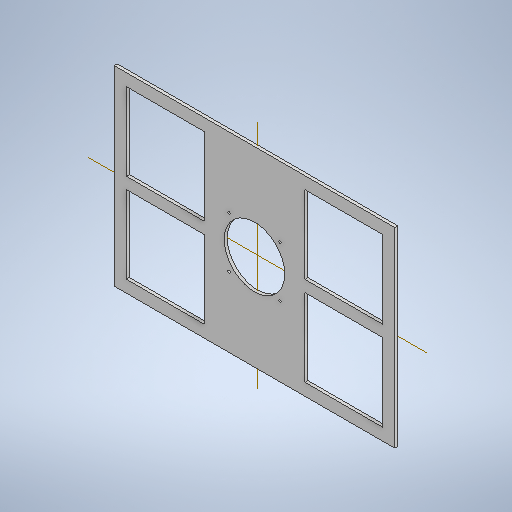
# Autodesk Inventor part: 가로세로
Saved by Autodesk Inventor 2025.1 (Build 291241000, 241)
## iProperties
Created: 2024-10-28
Part Number: 가로세로
Material: 일반
Document SubType Name: Modeling
Designer: gmsee
Density: 1 g/cm^3
Appearance: 기본값
Author: gmsee
Autodesk Inventor part; units mm, degrees
ref_plane "YZ Plane" through (0, 0, 0) normal (1, 0, 0) x (0, 1, 0)
ref_plane "XZ Plane" through (0, 0, 0) normal (0, 1, 0) x (-1, 0, 0)
ref_plane "XY Plane" through (0, 0, 0) normal (0, 0, 1) x (1, 0, 0)
sketch "스케치3" plane through (0, 0, 0) normal (0, 0, 1) x (1, 0, 0)
  line L0 (-232, 158) -> (232, 158)
  line L1 (232, 158) -> (232, -158)
  line L2 (232, -158) -> (-232, -158)
  line L3 (-232, -158) -> (-232, 158)
  line L4 (-212, -9.5) -> (-83.5, -9.5)
  line L5 (-83.5, -9.5) -> (-83.5, -138)
  line L6 (-83.5, -138) -> (-212, -138)
  line L7 (-212, -138) -> (-212, -9.5)
  line L8 (-212, 138) -> (-83.5, 138)
  line L9 (-83.5, 138) -> (-83.5, 9.5)
  line L10 (-83.5, 9.5) -> (-212, 9.5)
  line L11 (-212, 9.5) -> (-212, 138)
  line L12 (212, 138) -> (83.5, 138)
  line L13 (83.5, 138) -> (83.5, 9.5)
  line L14 (83.5, 9.5) -> (212, 9.5)
  line L15 (212, 9.5) -> (212, 138)
  line L16 (212, -138) -> (83.5, -138)
  line L17 (83.5, -138) -> (83.5, -9.5)
  line L18 (83.5, -9.5) -> (212, -9.5)
  line L19 (212, -9.5) -> (212, -138)
  circle A0 centre (-42.072, 42.072) radius 2
  circle A1 centre (42.072, 42.072) radius 2
  circle A2 centre (-42.072, -42.072) radius 2
  circle A3 centre (42.072, -42.072) radius 2
  line L20 (0, -221.2) -> (0, 221.2) projected
  line L21 (-324.8, 0) -> (324.8, 0) projected
  circle A4 centre (0, 0) radius 50
  point P0 (232, 0)
  point P1 (212, 73.75)
  dimension "d0" = 316
  dimension "d1" = 464
  dimension "d2" = 232
  dimension "d3" = 158
  dimension "d4" = 128.5
  dimension "d5" = 128.5
  dimension "d6" = 20
  dimension "d7" = 20
  dimension "d8" = 128.5
  dimension "d9" = 128.5
  dimension "d10" = 20
  dimension "d11" = 20
  dimension "d12" = 128.5
  dimension "d13" = 128.5
  dimension "d14" = 20
  dimension "d15" = 128.5
  dimension "d16" = 128.5
  dimension "d17" = 20
  dimension "d18" = 20
  dimension "d19" = 4
  dimension "d20" = 4
  dimension "d21" = 4
  dimension "d22" = 4
  dimension "d23" = 42.072
  dimension "d24" = 42.072
  dimension "d25" = 42.072
  dimension "d26" = 42.072
  dimension "d27" = 42.072
  dimension "d28" = 42.072
  dimension "d29" = 42.072
  dimension "d30" = 42.072
  dimension "d31" = 100
  constraints: 40 end point, 10 parallel, 5 centre point, 5 horizontal, 5 perpendicular, 2 midpoint, 1 coincident, 1 point on line
  measures "d0" distance of L0.end L1.end
  measures "d1" distance of L0.start L0.end
  measures "d2" distance of point (232, 0) point (0, 0)
  measures "d3" distance from line of L0 point (0, 0)
  measures "d4" distance of L4.end L5.end
  measures "d5" distance of L4.start L4.end
  measures "d6" distance between parallel lines of L2 L6
  measures "d7" distance between parallel lines of L3 L7
  measures "d8" distance between parallel lines of L9 L11
  measures "d9" distance between parallel lines of L10 L8
  measures "d10" distance between parallel lines of L0 L8
  measures "d11" distance between parallel lines of L3 L11
  measures "d12" distance between parallel lines of L14 L12
  measures "d13" distance between parallel lines of L15 L13
  measures "d14" distance from line of L1 point (212, 73.75)
  measures "d15" distance between parallel lines of L19 L17
  measures "d16" distance between parallel lines of L16 L18
  measures "d17" distance between parallel lines of L1 L19
  measures "d18" distance between parallel lines of L2 L16
  measures "d19" diameter of A0
  measures "d20" diameter of A1
  measures "d21" diameter of A2
  measures "d22" diameter of A3
  measures "d23" distance from line of L20 A0.centre
  measures "d24" distance from line of L20 A1.centre
  measures "d25" distance from line of L20 A2.centre
  measures "d26" distance from line of L20 A3.centre
  measures "d27" distance from line of L21 A2.centre
  measures "d28" distance from line of L21 A0.centre
  measures "d29" distance from line of L21 A1.centre
  measures "d30" distance from line of L21 A3.centre
  measures "d31" diameter of A4
extrude "돌출1" add sketch "스케치3" along normal blind 5 contours L0 L20 A4 L21 L3 | L0 L1 L21 A4 L20 | L21 A4 L20 L2 L3 | L1 L2 L20 A4 L21
